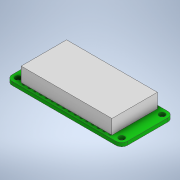
# Autodesk Inventor part: ESP8266 Feather
Saved by Autodesk Inventor 2021 (Build 250183000, 183)
## iProperties
Created: 2022-02-21
Part Number: ESP8266 Feather
Material: Generic
Document SubType Name: Modeling
Designer: maxsm
Density: 1 g/cm^3
Appearance: Default
Author: maxsm
Autodesk Inventor part; units mm, degrees
ref_plane "YZ Plane" through (0, 0, 0) normal (1, 0, 0) x (0, 1, 0)
ref_plane "XZ Plane" through (0, 0, 0) normal (0, 1, 0) x (-1, 0, 0)
ref_plane "XY Plane" through (0, 0, 0) normal (0, 0, 1) x (1, 0, 0)
sketch "Sketch1" plane through (0, 0, 0) normal (0, 1, 0) x (-1, 0, 0)
  line L0 (22.86, 11.43) -> (-22.86, 11.43)
  line L1 (-25.4, 8.89) -> (-25.4, -8.89)
  line L2 (-22.86, -11.43) -> (22.86, -11.43)
  line L3 (25.4, -8.89) -> (25.4, 8.89)
  line L4 (25.4, 11.43) -> (-25.4, -11.43) construction
  line L5 (-25.4, 11.43) -> (25.4, -11.43) construction
  circle A0 centre (22.86, 8.89) radius 1.27
  circle A1 centre (22.86, -8.89) radius 1.27
  circle A2 centre (-22.86, 8.89) radius 1.27
  circle A3 centre (-22.86, -8.89) radius 1.27
  arc A4 (25.4, 8.89) -> (22.86, 11.43) centre (22.86, 8.89) ccw
  arc A5 (22.86, -11.43) -> (25.4, -8.89) centre (22.86, -8.89) ccw
  arc A6 (-22.86, 11.43) -> (-25.4, 8.89) centre (-22.86, 8.89) ccw
  arc A7 (-25.4, -8.89) -> (-22.86, -11.43) centre (-22.86, -8.89) ccw
  point P0 (0, 0)
  dimension "d0" = 50.8
  dimension "d1" = 22.86
  dimension "d2" = 2.54
  dimension "d6" = 17.78
  dimension "d9" = 8.89
  dimension "d10" = 2.54
  dimension "d11" = 2.54
  dimension "d13" = 2.54
  dimension "d14" = 2.54
  dimension "d15" = 2.54
  constraints: 12 end point, 8 centre point, 8 point on circle, 8 point on line, 8 tangent, 6 equal radius, 2 horizontal alignment, 2 midpoint, 2 parallel, 1 horizontal, 1 perpendicular
  measures "d0" distance of L5.end L4.end
  measures "d1" distance of L4.end L5.start
  measures "d2" diameter of A0
  measures "d6" distance of A1.centre A0.centre
  measures "d9" vertical distance of A0.centre point (0, 0)
  measures "d10" distance from line of A0.centre L3
  measures "d11" distance from line of L3 A1.centre
  measures "d13" distance from line of L1 A3.centre
  measures "d14" distance from line of L1 A2.centre
  measures "d15" radius of A4
extrude "Extrusion1" add sketch "Sketch1" along normal blind 1.6
sketch "Sketch6" plane through (0, 1.6, 0) normal (0, 1, 0) x (1, 0, 0)
  circle A0 centre (-1.27, -10.16) radius 0.5
  line L0 (-22.86, -11.43) -> (22.86, -11.43) projected
  point P0 (0, 0)
  dimension "d46" = 1
  dimension "d47" = 1.27
  dimension "d48" = 1.27
  constraints: 1 centre point
  measures "d46" diameter of A0
  measures "d47" horizontal distance of A0.centre point (0, 0)
  measures "d48" distance from line of L0 A0.centre
extrude "Extrusion6" cut sketch "Sketch6" against normal through all
pattern_linear "Rectangular Pattern1" count 16 spacing 2.54 along (1, 0, 0) of "Extrusion6" first direction both ways yes
sketch "Sketch7" plane through (0, 1.6, 0) normal (0, 1, 0) x (1, 0, 0)
  circle A0 centre (3.81, 10.16) radius 0.5
  line L0 (-25.4, 8.89) -> (-25.4, -8.89) projected
  line L1 (22.86, 11.43) -> (-22.86, 11.43) projected
  point P0 (0, 0)
  point P1 (-25.4, 4.445)
  point P2 (-10.668, 11.43)
  dimension "d54" = 29.21
  dimension "d55" = 1.27
  dimension "d56" = 1
  constraints: 1 centre point
  measures "d54" distance from line of L0 A0.centre
  measures "d55" distance from line of L1 A0.centre
  measures "d56" diameter of A0
extrude "Extrusion7" cut sketch "Sketch7" against normal through all
pattern_linear "Rectangular Pattern2" count 12 spacing 2.54 along (1, 0, 0) of "Extrusion7" first direction both ways yes
sketch "Sketch11" plane through (0, 1.6, 0) normal (0, 1, 0) x (1, 0, 0)
  line L0 (-20.32, 10) -> (19.68, 10)
  line L1 (19.68, 10) -> (19.68, -10)
  line L2 (19.68, -10) -> (-20.32, -10)
  line L3 (-20.32, -10) -> (-20.32, 10)
  line L4 (-20.32, 10) -> (19.68, -10) construction
  line L5 (19.68, 10) -> (-20.32, -10) construction
  line L6 (-25.4, 8.89) -> (-25.4, -8.89) projected
  point P0 (0, 0)
  point P1 (-0.32, 0)
  point P2 (-0.32, 0)
  dimension "d77" = 40
  dimension "d78" = 20
  dimension "d81" = 5.08
  constraints: 12 end point, 3 midpoint, 2 parallel, 1 horizontal, 1 horizontal alignment, 1 perpendicular
  measures "d77" distance of L1.end L2.end
  measures "d78" distance of L0.end L1.end
  measures "d81" distance between parallel lines of L6 L3
extrude "Extrusion11" add sketch "Sketch11" along normal blind 6.35
body "Solid1"
